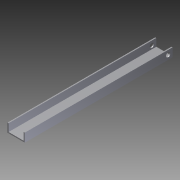
# Autodesk Inventor part: shooter U frame
Saved by Autodesk Inventor 2012 (Build 160160000, 160)
## iProperties
Created: 2013-07-07
Part Number: shooter U frame
Material: Default
Document SubType Name: Modeling
Designer: Bryce
Density: 1 g/cm^3
Author: Bryce
Autodesk Inventor part; units mm, degrees
ref_plane "YZ Plane" through (0, 0, 0) normal (1, 0, 0) x (0, 1, 0)
ref_plane "XZ Plane" through (0, 0, 0) normal (0, 1, 0) x (-1, 0, 0)
ref_plane "XY Plane" through (0, 0, 0) normal (0, 0, 1) x (1, 0, 0)
sketch "Sketch1" plane through (0, 0, 0) normal (0, 0, 1) x (1, 0, 0)
  line L0 (0, 0) -> (50.8, 0)
  line L1 (50.8, 0) -> (50.8, 25.4)
  line L2 (0, 25.4) -> (0, 0)
  line L3 (3.175, 3.175) -> (47.625, 3.175)
  line L4 (47.625, 3.175) -> (47.625, 25.4)
  line L5 (3.175, 25.4) -> (3.175, 3.175)
  line L6 (0, 25.4) -> (3.175, 25.4)
  line L7 (47.625, 25.4) -> (50.8, 25.4)
  dimension "d0" = 50.8
  dimension "d1" = 25.4
  dimension "d2" = 3.175
  dimension "d3" = 3.175
  dimension "d5" = 3.175
  constraints: 16 end point, 3 perpendicular, 2 horizontal, 2 parallel, 1 collinear
  measures "d0" distance of L1.end L2.start
  measures "d1" distance of L0.end L1.end
  measures "d2" distance between parallel lines of L2 L5
  measures "d3" distance between parallel lines of L0 L3
  measures "d5" distance between parallel lines of L1 L4
extrude "Extrusion1" add sketch "Sketch1" along normal blind 431.8
sketch "Sketch2" plane through (50.8, 0, 0) normal (1, 0, 0) x (0, 0, -1)
  line L0 (0, 0) -> (0, 25.4) projected
  line L1 (0, 25.4) -> (-431.8, 25.4) projected
  circle A0 centre (-12.7, 12.7) radius 6.35
  dimension "d8" = 12.7
  dimension "d9" = 12.7
  dimension "d10" = 12.7
  constraints: 1 centre point
  measures "d8" diameter of A0
  measures "d9" distance from line of L0 A0.centre
  measures "d10" distance from line of L1 A0.centre
extrude "Extrusion2" cut sketch "Sketch2" against normal blind 431.8
equation "\"d2\" = d5"
equation "\"d5\" = d4"
equation "\"d4\" = d3"
body "Solid1"
